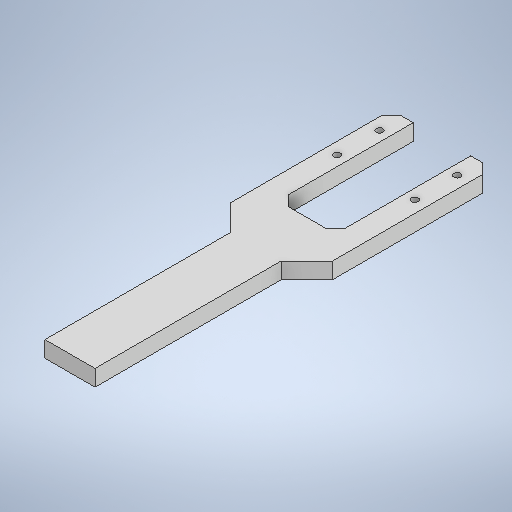
# Autodesk Inventor part: camera_holder
Saved by Autodesk Inventor 2027 (Build 310192060, 192F)
## iProperties
Created: 2026-05-27
Part Number: camera_holder
Material: Generic
Document SubType Name: Modeling
Designer: savas
Density: 1 g/cm^3
Appearance: Default
Author: savas
Autodesk Inventor part; units mm, degrees
ref_plane "YZ Plane" through (0, 0, 0) normal (1, 0, 0) x (0, 1, 0)
ref_plane "XZ Plane" through (0, 0, 0) normal (0, 1, 0) x (-1, 0, 0)
ref_plane "XY Plane" through (0, 0, 0) normal (0, 0, 1) x (1, 0, 0)
sketch "Sketch1" plane through (0, 0, 0) normal (0, 1, 0) x (-1, 0, 0)
  line L0 (0, 0) -> (30, 0)
  line L1 (30, 0) -> (30, -110)
  line L2 (30, -110) -> (0, -110)
  line L3 (0, -110) -> (0, 0)
  line L4 (6.5, -110) -> (23.5, -110)
  line L5 (23.5, -110) -> (23.5, -70)
  line L6 (23.5, -70) -> (6.5, -70)
  line L7 (6.5, -70) -> (6.5, -110)
  circle A0 centre (26.5, -103) radius 1
  circle A1 centre (3.5, -103) radius 1
  line L8 (30, -105) -> (0, -105) construction
  circle A2 centre (26.5, -90.5) radius 1
  circle A3 centre (3.5, -90.5) radius 1
  line L9 (22.4, 0) -> (7.6, 0)
  line L10 (7.6, 0) -> (7.6, -55)
  line L11 (7.6, -55) -> (22.4, -55)
  line L12 (22.4, -55) -> (22.4, 0)
  line L13 (22.4, -55) -> (30, -62.6)
  line L14 (22.4, -55) -> (33.148, -55) construction
  line L15 (7.6, -55) -> (0, -62.6)
  line L16 (7.6, -55) -> (18.348, -55) construction
  point P0 (27.5, -90.5)
  point P1 (2.5, -90.5)
  point P2 (15, 0)
  point P3 (15, -55)
  point P4 (15, -70)
  point P5 (22.4, 0)
  point P6 (7.6, 0)
  dimension "d0" = 30
  dimension "d1" = 110
  dimension "d2" = 2
  dimension "d3" = 2
  dimension "d4" = 14.5
  dimension "d5" = 5
  dimension "d6" = 25
  dimension "d7" = 3
  dimension "d8" = 3
  dimension "d11" = 3.5
  dimension "d12" = 3.5
  dimension "d13" = 40
  dimension "d19" = 14.8
  dimension "d20" = 55
  dimension "d21" = 45
  dimension "d22" = 135
  constraints: 34 end point, 6 parallel, 5 horizontal, 5 horizontal alignment, 5 point on line, 4 perpendicular, 3 midpoint, 3 vertical alignment, 2 centre point, 2 equal length, 1 equal radius, 6 other
  measures "d0" distance of L1.end L2.end
  measures "d1" distance of L0.end L1.end
  measures "d2" diameter of A0
  measures "d3" distance from line of L8 A0.centre
  measures "d4" distance from line of L8 point (26.5, -90.5)
  measures "d5" distance between parallel lines of L2 L8
  measures "d6" distance of point (2.5, -90.5) point (27.5, -90.5)
  measures "d7" distance from line of L5 point (26.5, -90.5)
  measures "d8" distance from line of L7 point (3.5, -90.5)
  measures "d11" distance from line of L3 point (3.5, -90.5)
  measures "d12" distance from line of L1 point (26.5, -90.5)
  measures "d13" distance between parallel lines of L4 L6
  measures "d19" distance of L11.end L10.end
  measures "d20" distance of L10.end L9.end
  measures "d21" angle of L13 L14
  measures "d22" angle of L15 L16
extrude "Extrusion1" add sketch "Sketch1" along normal blind 4.8 contours L0 L12 L11 L10 | L15 L11 L13 L1 L2 L5 L6 L7 L3
chamfer "Chamfer1" distance 3 angle 45 4 edges at (-23.5, 2.4, -70) (-6.5, 2.4, -70) (-30, 2.4, -110) (0, 2.4, -110)
body "Solid1"
